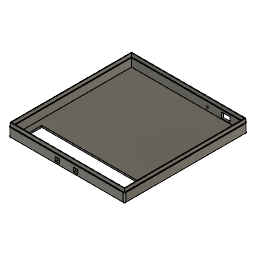
Casing Top (Autodesk Fusion 360 design; units mm, degrees)
part number: 2026-02-02-17-51-03-125
Autodesk Fusion 360 part; units mm, degrees
sketch "Sketch1" plane through (0, 0, 0) normal (0, 0, 1) x (1, 0, 0)
  line L0 (2, 0) -> (162, 0)
  line L1 (164, 2) -> (164, 172)
  line L2 (162, 174) -> (2, 174)
  line L3 (0, 172) -> (0, 2)
  arc A0 (2, 174) -> (0, 172) centre (2, 172) ccw
  arc A1 (164, 172) -> (162, 174) centre (162, 172) ccw
  arc A2 (0, 2) -> (2, 0) centre (2, 2) ccw
  arc A3 (162, 0) -> (164, 2) centre (162, 2) ccw
  point P0 (164, 0)
  point P1 (0, 174)
  dimension "d1" = 164
  dimension "d2" = 174
  dimension "d3" = 2
  dimension "d4" = 2
  dimension "d5" = 2
  dimension "d6" = 2
  constraint horizontal L0
  constraint vertical L1
  constraint horizontal L2
  constraint vertical L3
  constraint coincident P1 L2
  constraint coincident P1 L3
  constraint tangent L2 A0
  constraint tangent L3 A0
  constraint tangent L2 A1
  constraint tangent L1 A1
  constraint coincident origin L3
  constraint coincident origin L0
  constraint tangent L3 A2
  constraint tangent L0 A2
  constraint coincident P0 L1
  constraint coincident P0 L0
  constraint tangent L1 A3
  constraint tangent L0 A3
  measures "d1" distance of origin P0
  measures "d2" distance of origin P1
  measures "d3" radius of A0
  measures "d4" radius of A1
  measures "d5" radius of A2
  measures "d6" radius of A3
extrude "Extrude1" add sketch "Sketch1" along normal blind 14
sketch "Sketch4" plane through (0, 0, 14) normal (0, 0, 1) x (-1, 0, 0)
  arc A0 (-162, 0) -> (-164, -2) centre (-162, -2) ccw
  line L0 (-164, -2) -> (-164, -172)
  arc A1 (-164, -172) -> (-162, -174) centre (-162, -172) ccw
  line L1 (-162, -174) -> (-2, -174)
  arc A2 (-2, -174) -> (0, -172) centre (-2, -172) ccw
  line L2 (0, -172) -> (0, -2)
  arc A3 (0, -2) -> (-2, 0) centre (-2, -2) ccw
  line L3 (-2, 0) -> (-162, 0)
  line L4 (-1.1, -172.9) -> (-162.9, -172.9)
  line L5 (-162.9, -172.9) -> (-162.9, -1.1)
  line L6 (-162.9, -1.1) -> (-1.1, -1.1)
  line L7 (-1.1, -1.1) -> (-1.1, -172.9)
  dimension "d19" = 161.8
  dimension "d20" = 171.8
  dimension "d21" = 1.1
  dimension "d22" = 1.1
  constraint horizontal L4
  constraint vertical L5
  constraint horizontal L6
  constraint vertical L7
  measures "d19" distance of L4.start L4.end
  measures "d20" distance of L4.start L6.end
  measures "d21" distance of L1 L4
  measures "d22" distance of L2 L7
extrude "Extrude4" add sketch "Sketch4" along normal blind 5 contours L4 L5 L6 L7
sketch "Sketch5" plane through (0, 0, 19) normal (0, 0, 1) x (-1, 0, 0)
  line L0 (-1.1, -1.1) -> (-162.9, -1.1)
  line L1 (-162.9, -1.1) -> (-162.9, -172.9)
  line L2 (-162.9, -172.9) -> (-1.1, -172.9)
  line L3 (-1.1, -172.9) -> (-1.1, -1.1)
  line L4 (-1.9, -172.1) -> (-162.1, -172.1)
  line L5 (-162.1, -172.1) -> (-162.1, -1.9)
  line L6 (-162.1, -1.9) -> (-1.9, -1.9)
  line L7 (-1.9, -1.9) -> (-1.9, -172.1)
  dimension "d25" = 160.2
  dimension "d26" = 170.2
  dimension "d27" = 0.8
  dimension "d28" = 0.8
  constraint horizontal L4
  constraint vertical L5
  constraint horizontal L6
  constraint vertical L7
  measures "d25" distance of L4.start L4.end
  measures "d26" distance of L4.start L6.end
  measures "d27" distance of L3 L7
  measures "d28" distance of L2 L4
extrude "Extrude5" cut sketch "Sketch5" against normal blind 5 contours L4 L5 L6 L7
sketch "Sketch6" plane through (0, 0, 14) normal (0, 0, 1) x (-1, 0, 0)
  line L0 (-1.9, -1.9) -> (-162.1, -1.9)
  line L1 (-162.1, -1.9) -> (-162.1, -172.1)
  line L2 (-162.1, -172.1) -> (-1.9, -172.1)
  line L3 (-1.9, -172.1) -> (-1.9, -1.9)
  line L4 (-2.9, -171.1) -> (-160.9, -171.1)
  line L5 (-160.9, -171.1) -> (-160.9, -3.1)
  line L6 (-160.9, -3.1) -> (-2.9, -3.1)
  line L7 (-2.9, -3.1) -> (-2.9, -171.1)
  dimension "d31" = 158
  dimension "d32" = 168
  dimension "d33" = 1
  dimension "d34" = 1
  constraint horizontal L4
  constraint vertical L5
  constraint horizontal L6
  constraint vertical L7
  measures "d31" distance of L4.start L4.end
  measures "d32" distance of L4.start L6.end
  measures "d33" distance of L3 L7
  measures "d34" distance of L2 L4
extrude "Extrude6" cut sketch "Sketch6" against normal blind 11.5 contours L4 L5 L6 L7
sketch "Sketch9" plane through (0, 0, 2.5) normal (0, 0, 1) x (-1, 0, 0)
  line L0 (-2.9, -3.1) -> (-160.9, -3.1)
  line L1 (-160.9, -3.1) -> (-160.9, -171.1)
  line L2 (-160.9, -171.1) -> (-2.9, -171.1)
  line L3 (-2.9, -171.1) -> (-2.9, -3.1)
  line L4 (-10.9, -16.1) -> (-147.9, -16.1)
  line L5 (-147.9, -16.1) -> (-147.9, -36.1)
  line L6 (-147.9, -36.1) -> (-10.9, -36.1)
  line L7 (-10.9, -36.1) -> (-10.9, -16.1)
  dimension "d37" = 137
  dimension "d38" = 20
  dimension "d39" = 13
  dimension "d40" = 8
  constraint horizontal L4
  constraint vertical L5
  constraint horizontal L6
  constraint vertical L7
  measures "d37" distance of L4.start L4.end
  measures "d38" distance of L4.start L6.end
  measures "d39" distance of L0 L4
  measures "d40" distance of L3 L7
extrude "Extrude7" cut sketch "Sketch9" against normal blind 2.5 contours L4 L5 L6 L7
sketch "Sketch10" plane through (0, 0, 0) normal (0, -1, 0) x (1, 0, 0)
  line L0 (2, 0) -> (162, 0)
  line L1 (162, 0) -> (162, 14)
  line L2 (162, 14) -> (2, 14)
  line L3 (2, 14) -> (2, 0)
  line L4 (66, 10) -> (72, 10)
  line L5 (72, 10) -> (72, 4)
  line L6 (72, 4) -> (66, 4)
  line L7 (66, 4) -> (66, 10)
  dimension "d43" = 6
  dimension "d44" = 6
  dimension "d45" = 4
  dimension "d46" = 64
  constraint horizontal L4
  constraint vertical L5
  constraint horizontal L6
  constraint vertical L7
  measures "d43" distance of L4.start L4.end
  measures "d44" distance of L4.start L6.end
  measures "d45" distance of L2 L4
  measures "d46" distance of L3 L7
sketch "Sketch11" plane through (0, 0, 0) normal (0, -1, 0) x (1, 0, 0)
  line L0 (92, 10) -> (98, 10)
  line L1 (98, 10) -> (98, 4)
  line L2 (98, 4) -> (92, 4)
  line L3 (92, 4) -> (92, 10)
  line L4 (162, 14) -> (2, 14)
  line L5 (162, 0) -> (162, 14)
  dimension "d47" = 6
  dimension "d48" = 6
  dimension "d49" = 4
  dimension "d50" = 64
  constraint horizontal L0
  constraint vertical L1
  constraint horizontal L2
  constraint vertical L3
  measures "d47" distance of L0.start L0.end
  measures "d48" distance of L0.start L2.end
  measures "d49" distance of L0 L4
  measures "d50" distance of L1 L5
extrude "Extrude8" cut sketch "Sketch10" against normal blind 3 contours L4 L5 L6 L7
extrude "Extrude9" cut sketch "Sketch11" against normal blind 3
sketch "Sketch12" plane through (0, 174, 0) normal (0, 1, 0) x (-1, 0, 0)
  line L0 (-162, 0) -> (-2, 0)
  line L1 (-2, 0) -> (-2, 14)
  line L2 (-2, 14) -> (-162, 14)
  line L3 (-162, 14) -> (-162, 0)
  line L4 (-142, 11) -> (-130, 11)
  line L5 (-130, 11) -> (-130, 3)
  line L6 (-130, 3) -> (-142, 3)
  line L7 (-142, 3) -> (-142, 11)
  dimension "d55" = 12
  dimension "d56" = 8
  dimension "d57" = 20
  dimension "d58" = 3
  constraint horizontal L4
  constraint vertical L5
  constraint horizontal L6
  constraint vertical L7
  measures "d55" distance of L4.start L4.end
  measures "d56" distance of L4.start L6.end
  measures "d57" distance of L3 L7
  measures "d58" distance of L0 L6
sketch "Sketch13" plane through (0, 174, 0) normal (0, 1, 0) x (-1, 0, 0)
  circle A0 centre (-110, 7) radius 1.5
  line L0 (-130, 11) -> (-130, 3)
  line L1 (-2, 14) -> (-162, 14)
  dimension "d59" = 3
  dimension "d60" = 20
  dimension "d61" = 7
  measures "d59" diameter of A0
  measures "d60" distance of A0.centre L0
  measures "d61" distance of A0.centre L1
extrude "Extrude10" cut sketch "Sketch12" against normal blind 3 contours L4 L5 L6 L7
extrude "Extrude11" cut sketch "Sketch13" against normal blind 3
fillet "Fillet1" radius 2 8 edges at (82, 174, 0) (0.5858, 173.4142, 0) (0, 87, 0) (0.5858, 0.5858, 0) (82, 0, 0) (163.4142, 0.5858, 0) (164, 87, 0) (163.4142, 173.4142, 0)
